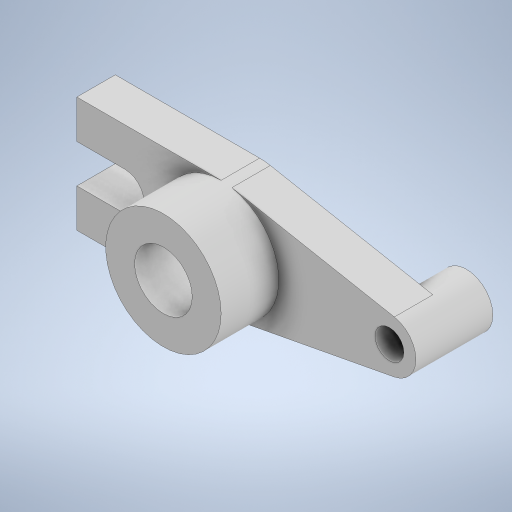
# Autodesk Inventor part: 05-08-2023 sfomatura
Saved by Autodesk Inventor 2023 (Build 270158000, 158)
## iProperties
Created: 2023-05-08
Part Number: 05-08-2023 sfomatura
Material: Generico
Document SubType Name: Modeling
Designer: Admin
Density: 1 g/cm^3
Appearance: Default
Author: Admin
Autodesk Inventor part; units mm, degrees
ref_plane "YZ Plane" through (0, 0, 0) normal (1, 0, 0) x (0, 1, 0)
ref_plane "XZ Plane" through (0, 0, 0) normal (0, 1, 0) x (-1, 0, 0)
ref_plane "XY Plane" through (0, 0, 0) normal (0, 0, 1) x (1, 0, 0)
sketch "Schizzo1" plane through (0, 0, 0) normal (0, 0, 1) x (1, 0, 0)
  circle A0 centre (0, 0) radius 12
  circle A1 centre (0, 0) radius 6
  circle A2 centre (35, 0) radius 5.5
  circle A3 centre (35, 0) radius 3
  line L0 (0, 0) -> (107.6608, 0) construction
  line L1 (0, 0) -> (107.6608, 0) construction
  line L2 (0, 12) -> (-30, 12)
  line L3 (-30, 12) -> (-30, 4)
  line L4 (-30, 4) -> (-20, 4)
  arc A4 (-20, -4) -> (-20, 4) centre (-20, 0) ccw
  line L5 (-20, -4) -> (-30, -4)
  line L6 (-30, -4) -> (-30, -12)
  line L7 (-30, -12) -> (0, -12)
  line L8 (2.2286, -11.7912) -> (36.0214, -5.4043)
  line L9 (2.2286, 11.7912) -> (36.0214, 5.4043)
  dimension "d1" = 10
  dimension "d2" = 12
  dimension "d3" = 24
  dimension "d4" = 4
  dimension "d5" = 8
  dimension "d6" = 8
  dimension "d7" = 30
  dimension "d8" = 35
  dimension "d9" = 11
  dimension "d10" = 6
  constraints: 20 end point, 8 point on circle, 8 tangent, 5 centre point, 4 perpendicular, 3 coincident, 3 equal length, 2 vertical, 1 horizontal, 1 point on line, 1 other
  measures "d1" distance of L3.end L4.end
  measures "d2" diameter of A1
  measures "d3" diameter of A0
  measures "d4" radius of A4
  measures "d5" distance of L2.end L3.end
  measures "d6" distance of L5.end L6.end
  measures "d7" distance of L2.start L2.end
  measures "d8" distance of point (0, 0) A2.centre
  measures "d9" diameter of A2
  measures "d10" diameter of A3
extrude "Estrusione1" add sketch "Schizzo1" along normal blind 3 and the other way blind 5
extrude "Estrusione2" add sketch "Schizzo1" against normal blind 13 contours A2
extrude "Estrusione3" add sketch "Schizzo1" along normal blind 15 contours A0
